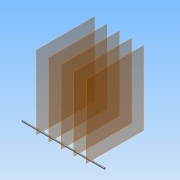
# Autodesk Inventor part: Selection_Selector Shaft
Saved by Autodesk Inventor 2018.1 (Build 221171000, 171)
## iProperties
Created: 2019-02-07
Part Number: Selection_Selector Shaft
Material: Steel, Mild
Document SubType Name: Modeling
Designer: James
Density: 7.85 g/cm^3
Appearance: Semi-Polished
Mass: 72.2727 g
Surface Area: 62.8406 cm^2
Volume: 9.20672 cm^3
Author: James
Autodesk Inventor part; units mm, degrees
ref_plane "YZ Plane" through (0, 0, 0) normal (1, 0, 0) x (0, 1, 0)
ref_plane "XZ Plane" through (0, 0, 0) normal (0, 1, 0) x (-1, 0, 0)
ref_plane "XY Plane" through (0, 0, 0) normal (0, 0, 1) x (1, 0, 0)
derived "Selection_Skeleton.ipt"
ref_plane "Ground" through (0, 0, 0) normal (0, 1, 0) x (-1, 0, 0)
ref_plane "LHS inner" through (0, 0, 0) normal (1, 0, 0) x (0, 1, 0)
ref_plane "RHS inner" through (300, 0, 0) normal (1, 0, 0) x (0, 1, 0)
ref_plane "Lane 1" through (50, 0, 0) normal (1, 0, 0) x (0, 1, 0)
ref_plane "Lane 2" through (100, 0, 0) normal (1, 0, 0) x (0, 1, 0)
ref_plane "Lane 3" through (150, 0, 0) normal (1, 0, 0) x (0, 1, 0)
ref_plane "Lane 4" through (200, 0, 0) normal (1, 0, 0) x (0, 1, 0)
ref_plane "Lane 5" through (250, 0, 0) normal (1, 0, 0) x (0, 1, 0)
ref_plane "Back" through (0, 0, 0) normal (0, 0, 1) x (1, 0, 0)
sketch "Sketch1" plane through (0, 0, 0) normal (1, 0, 0) x (0, 1, 0)
  circle A0 centre (0, 0) radius 3
  dimension "d1" = 6
  constraints: 1 centre point, 1 coincident
  measures "d1" diameter of A0
extrude "Extrusion1" add sketch "Sketch1" along normal up to surface (300 mm away)
ref_plane "Work Plane11" through (150, 0, 0) normal (1, 0, 0) x (0, 1, 0)
sketch "Sketch2" plane through (300, 0, 0) normal (1, 0, 0) x (0, 0, -1)
  circle A0 centre (0, 0) radius 3 projected
extrude "Weight side" add sketch "Sketch2" along normal blind 15
sketch "Sketch3" plane through (0, 0, 0) normal (-1, 0, 0) x (0, 0, 1)
  circle A0 centre (0, 0) radius 3 projected
extrude "Lever side" add sketch "Sketch3" along normal blind 17
sketch "Sketch4" plane through (0, 0, 0) normal (0, 0, 1) x (1, 0, 0)
  line L0 (40.8, 3) -> (40, 3)
  line L1 (40, 3) -> (40, 2.85)
  line L2 (40, 2.85) -> (40.8, 2.85)
  line L3 (40.8, 2.85) -> (40.8, 3)
  line L4 (63.8, 3) -> (63, 3)
  line L5 (63, 3) -> (63, 2.85)
  line L6 (63, 2.85) -> (63.8, 2.85)
  line L7 (63.8, 2.85) -> (63.8, 3)
  line L8 (-72.76, 0) -> (86.56, 0) projected
  line L9 (-17, 3) -> (-17, -3) projected
  line L10 (50, 4.2) -> (50, -4.2) projected
  point P0 (0, 0)
  dimension "d8" = 2.85
  dimension "d9" = 0.8
  dimension "d10" = 0.8
  dimension "d33" = 10
  dimension "d34" = 13
  constraints: 16 end point, 4 parallel, 3 horizontal alignment, 2 horizontal, 2 perpendicular, 2 point on line
  measures "d8" distance between parallel lines of L8 L2
  measures "d9" distance of L0.start L0.end
  measures "d10" distance of L4.start L4.end
  measures "d33" distance from line of L10 L0.end
  measures "d34" distance from line of L4.end L10
revolve "Revolution1" [suppressed]
pattern_linear "Rectangular Pattern1" [suppressed]
chamfer "Chamfer4" [suppressed]
sketch "Sketch6" plane through (0, 0, 0) normal (0, 0, 1) x (1, 0, 0)
  line L0 (15, 3) -> (15.8, 3)
  line L1 (15.8, 3) -> (15.8, 2.85)
  line L2 (15.8, 2.85) -> (15, 2.85)
  line L3 (15, 2.85) -> (15, 3)
  line L4 (-62.56, 0) -> (28.86, 0) projected
  line L5 (-16.5, 3) -> (-16.5, -3) projected
  line L6 (0, 4.2) -> (0, -4.2) projected
  point P0 (0, 0)
  dimension "d38" = 0.8
  dimension "d39" = 2.85
  dimension "d40" = 15
  constraints: 8 end point, 2 parallel, 1 horizontal, 1 horizontal alignment, 1 perpendicular
  measures "d38" distance of L0.start L0.end
  measures "d39" distance between parallel lines of L4 L2
  measures "d40" distance from line of L0.start L6
revolve "Revolution3" [suppressed]
mirror "Mirror2" [suppressed]
sketch "Sketch7" plane through (0, 0, 0) normal (0, 1, 0) x (-1, 0, 0)
  line L0 (-311.5, 3) -> (-315, 3)
  line L1 (-315, 3) -> (-315, 1.5)
  line L2 (-315, 1.5) -> (-311.5, 1.5)
  line L3 (-311.5, 1.5) -> (-311.5, 3)
  line L4 (-315, 3) -> (-315, -3) projected
  line L5 (123, 0) -> (-388, 0) projected
  point P0 (0, 0)
  point P1 (-285, 3)
  point P2 (-285, -3)
  dimension "d42" = 3.5
  dimension "d43" = 1.5
  constraints: 8 end point, 2 parallel, 1 coincident, 1 horizontal, 1 perpendicular, 1 point on line, 1 vertical alignment
  measures "d42" distance of L0.start L0.end
  measures "d43" distance between parallel lines of L5 L2
revolve "Revolution4" [suppressed]
chamfer "Chamfer5" [suppressed]
fillet "Fillet2" [suppressed]
ref_plane "Mid end planes" through (149, 0, 0) normal (-1, 0, 0) x (0, 0, 1)
mirror "Mirror3" [suppressed]
chamfer "Chamfer6" [suppressed]
equation "\"d10\" = d9"
body "Solid1"
